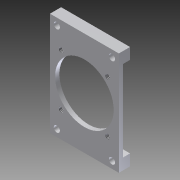
# Autodesk Inventor part: Dewalt CAP Clamp Plate
Saved by Autodesk Inventor 2012 (Build 160160000, 160)
## iProperties
Created: 2012-07-04
Part Number: Dewalt CAP Clamp Plate
Material: Default
Document SubType Name: Modeling
Designer: Bruce
Density: 1 g/cm^3
Author: Bruce
Autodesk Inventor part; units mm, degrees
ref_plane "YZ Plane" through (0, 0, 0) normal (1, 0, 0) x (0, 1, 0)
ref_plane "XZ Plane" through (0, 0, 0) normal (0, 1, 0) x (-1, 0, 0)
ref_plane "XY Plane" through (0, 0, 0) normal (0, 0, 1) x (1, 0, 0)
sketch "Sketch1" plane through (0, 0, 0) normal (0, 0, 1) x (1, 0, 0)
  line L0 (-25.4, 38.1) -> (25.4, 38.1)
  line L1 (25.4, 38.1) -> (25.4, -38.1)
  line L2 (25.4, -38.1) -> (-25.4, -38.1)
  line L3 (-25.4, -38.1) -> (-25.4, 38.1)
  circle A0 centre (0, 0) radius 21.59
  circle A1 centre (-20.32, 33.02) radius 2.286
  circle A2 centre (0, 0) radius 19.05 construction
  circle A3 centre (20.32, 33.02) radius 2.286
  circle A4 centre (-20.32, -33.02) radius 2.286
  circle A5 centre (20.32, -33.02) radius 2.286
  point P0 (-17.145, 19.05)
  point P1 (17.145, 19.05)
  point P2 (17.145, -19.05)
  point P3 (-17.145, -19.05)
  dimension "d0" = 43.18
  dimension "d1" = 76.2
  dimension "d2" = 38.1
  dimension "d3" = 50.8
  dimension "d4" = 25.4
  dimension "d5" = 4.572
  dimension "d6" = 5.08
  dimension "d7" = 5.08
  dimension "d8" = 38.1
  dimension "d9" = 4.572
  dimension "d10" = 5.08
  dimension "d11" = 5.08
  dimension "d12" = 4.572
  dimension "d13" = 4.572
  dimension "d20" = 66.04
  dimension "d21" = 40.64
  dimension "d23" = 34.29
  dimension "d24" = 19.05
  dimension "d25" = 19.05
  dimension "d26" = 17.145
  constraints: 8 end point, 6 centre point, 4 horizontal alignment, 4 vertical alignment, 2 coincident, 2 parallel, 1 horizontal, 1 perpendicular
  measures "d0" diameter of A0
  measures "d1" distance of L2.end L0.start
  measures "d2" distance from line of L0 point (0, 0)
  measures "d3" distance of L0.start L0.end
  measures "d4" distance from line of L3 point (0, 0)
  measures "d5" diameter of A1
  measures "d6" distance from line of A1.centre L0
  measures "d7" distance from line of L3 A1.centre
  measures "d8" diameter of A2
  measures "d9" diameter of A3
  measures "d10" distance from line of L1 A3.centre
  measures "d11" distance from line of L2 A4.centre
  measures "d12" diameter of A4
  measures "d13" diameter of A5
  measures "d20" distance of A4.centre A1.centre
  measures "d21" distance of A5.centre A4.centre
  measures "d23" distance of point (17.145, 19.05) point (-17.145, 19.05)
  measures "d24" vertical distance of point (0, 0) point (-17.145, 19.05)
  measures "d25" vertical distance of point (-17.145, -19.05) point (0, 0)
  measures "d26" horizontal distance of point (-17.145, 19.05) A2.centre
extrude "Extrusion1" add sketch "Sketch1" against normal blind 3.175
sketch "Sketch2" plane through (0, 0, -3.175) normal (0, 0, -1) x (-1, 0, 0)
  circle A0 centre (-20.32, -33.02) radius 2.286 projected
  circle A1 centre (20.32, -33.02) radius 2.286 projected
  circle A2 centre (-20.32, 33.02) radius 2.286 projected
  circle A3 centre (20.32, 33.02) radius 2.286 projected
  line L0 (25.4, 38.1) -> (25.4, -38.1) projected
  line L1 (-25.4, 38.1) -> (25.4, 38.1) projected
  line L2 (-25.4, -38.1) -> (-25.4, 38.1) projected
  line L3 (25.4, -38.1) -> (-25.4, -38.1) projected
  line L4 (-25.4, 38.1) -> (25.4, 38.1)
  line L5 (25.4, 38.1) -> (25.4, 29.845)
  line L6 (25.4, 29.845) -> (-25.4, 29.845)
  line L7 (-25.4, 29.845) -> (-25.4, 38.1)
  line L8 (-25.4, -38.1) -> (25.4, -38.1)
  line L9 (25.4, -38.1) -> (25.4, -29.845)
  line L10 (25.4, -29.845) -> (-25.4, -29.845)
  line L11 (-25.4, -29.845) -> (-25.4, -38.1)
  dimension "d16" = 8.255
  dimension "d17" = 8.255
  constraints: 16 end point, 4 parallel, 3 collinear, 3 point on line, 2 horizontal, 2 perpendicular
  measures "d16" distance between parallel lines of L6 L1
  measures "d17" distance between parallel lines of L3 L10
extrude "Extrusion2" add sketch "Sketch2" along normal blind 5.08 contours L0 L6 L2 L1 | L0 L3 L2 L10
hole "Hole1" at (-17.145, 19.05, 0) at (17.145, 19.05, 0) at (17.145, -19.05, 0) at (-17.145, -19.05, 0) direction (0, 0, -1) diameter 3.302 end through all thread size "8-32 UNC" class "2B" standard "ANSI Unified Screw Threads"
equation "\"d2\" = 0.5 * d1"
equation "\"d4\" = 0.5 * d3"
equation "\"d9\" = d5"
equation "\"d12\" = d5"
equation "\"d13\" = d5"
equation "\"d26\" = 0.5 * d23"
equation "\"d17\" = d16"
body "Solid1"
